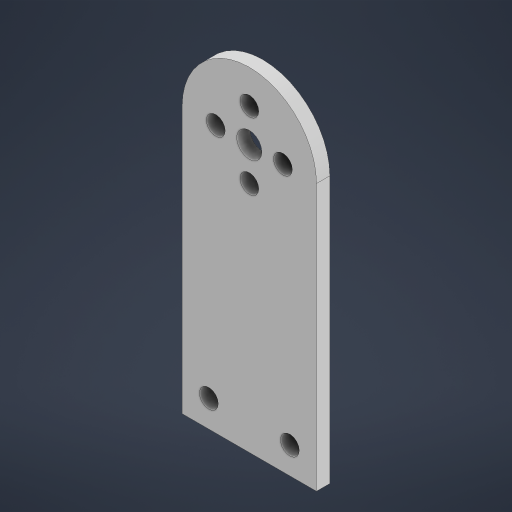
# Autodesk Inventor part: New_Wrist
Saved by Autodesk Inventor 2023 (Build 270158000, 158)
## iProperties
Created: 2024-02-19
Part Number: New_Wrist
Material: Generic
Document SubType Name: Modeling
Designer: kelle
Density: 1 g/cm^3
Appearance: Default
Author: kelle
Autodesk Inventor part; units mm, degrees
ref_plane "YZ Plane" through (0, 0, 0) normal (1, 0, 0) x (0, 1, 0)
ref_plane "XZ Plane" through (0, 0, 0) normal (0, 1, 0) x (-1, 0, 0)
ref_plane "XY Plane" through (0, 0, 0) normal (0, 0, 1) x (1, 0, 0)
sketch "Sketch1" plane through (0, 0, 0) normal (0, 0, 1) x (1, 0, 0)
  circle A0 centre (0, 0) radius 3
  circle A1 centre (0, 8) radius 2.25
  circle A2 centre (-8, 0) radius 2.25
  circle A3 centre (0, -8) radius 2.25
  circle A4 centre (8, 0) radius 2.25
  circle A5 centre (0, 0) radius 16
  line L0 (-16, 0) -> (-16, -63.5)
  line L1 (16, 0) -> (16, -63.5)
  line L2 (16, -63.5) -> (-16, -63.5)
  line L3 (0, -63.5) -> (0, 16) construction
  circle A6 centre (-9.65, -57.15) radius 2.25
  circle A7 centre (9.65, -57.15) radius 2.25
  point P0 (-16, -31.75)
  dimension "d0" = 6
  dimension "d1" = 4.5
  dimension "d2" = 8
  dimension "d5" = 360
  dimension "d7" = 32
  dimension "d8" = 63.5
  dimension "d9" = 32
  dimension "d10" = 4.5
  dimension "d11" = 4.5
  dimension "d12" = 6.35
  dimension "d13" = 6.35
  dimension "d14" = 6.35
  dimension "d15" = 6.35
  dimension "d16" = 19.3
  constraints: 8 centre point, 8 end point, 3 point on circle, 3 vertical, 2 coincident, 2 midpoint, 1 perpendicular, 1 tangent, 9 other
  measures "d0" diameter of A0
  measures "d1" diameter of A1
  measures "d2" distance of point (0, 0) A1.centre
  measures "d7" diameter of A5
  measures "d8" distance of L0.start L0.end
  measures "d9" distance from line of point (-16, -31.75) L1
  measures "d10" diameter of A6
  measures "d11" diameter of A7
  measures "d12" distance from line of L1 A7.centre
  measures "d13" distance from line of L2 A7.centre
  measures "d14" distance from line of L2 A6.centre
  measures "d15" distance from line of L0 A6.centre
  measures "d16" distance of A7.centre A6.centre
extrude "Extrusion1" add sketch "Sketch1" along normal blind 3.175
body "Solid1"
